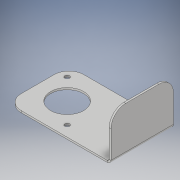
# Autodesk Inventor part: frontMotorMount
Saved by Autodesk Inventor 2017 (Build 210142000, 142)
## iProperties
Created: 2017-03-21
Part Number: frontMotorMount
Material: Generic
Document SubType Name: Sheet Metal
Designer: kingb
Density: 1 g/cm^3
Sheet Metal Rule: Default
Appearance: Default
Flat Pattern Width: 5.3975 cm
Flat Pattern Length: 12.7 cm
Flat Pattern Area: 68.5482 cm^2
Sheet Metal Width: 2.125 in
Sheet Metal Length: 5.000 in
Sheet Metal Area: 10.625 in^2
Author: kingb
Autodesk Inventor part; units mm, degrees
ref_plane "YZ Plane" through (0, 0, 0) normal (1, 0, 0) x (0, 1, 0)
ref_plane "XZ Plane" through (0, 0, 0) normal (0, 1, 0) x (-1, 0, 0)
ref_plane "XY Plane" through (0, 0, 0) normal (0, 0, 1) x (1, 0, 0)
sketch "Sketch1" plane through (0, 0, 0) normal (0, 1, 0) x (-1, 0, 0)
  line L0 (0, 0) -> (127, 0)
  line L1 (127, 0) -> (127, -53.975)
  line L2 (127, -53.975) -> (0, -53.975)
  line L3 (0, -53.975) -> (0, 0)
  line L4 (38.1, -53.975) -> (38.1, 0) construction
  line L5 (38.1, -26.9875) -> (101.6, -26.9875) construction
  circle A0 centre (101.6, -26.9875) radius 14.2875
  dimension "d0" = 127
  dimension "d1" = 53.975
  dimension "d2" = 38.1
  dimension "d3" = 63.5
  dimension "d4" = 28.575
  measures "d0" distance of L1.end L2.end
  measures "d1" distance of L0.end L1.end
  measures "d2" distance between parallel lines of L3 L4
  measures "d3" distance of L5.start L5.end
  measures "d4" diameter of A0
extrude "Plate1" add sketch "Sketch1" along normal blind 1.5875
fillet "Corner Round1" radius 12.7 2 edges at (-127, 0.7937, -53.975) (-127, 0.7937, 0)
fillet "Corner Round2" radius 12.7 2 edges at (0, 0.7937, 0) (0, 0.7937, -53.975)
sketch "Sketch2" plane through (0, 1.5875, 0) normal (0, 1, 0) x (1, 0, 0)
  circle A0 centre (-83.6395, 9.027) radius 2.0193 projected
  circle A1 centre (-119.5605, 44.948) radius 2.0193 projected
  point P0 (0, 0)
extrude "Extrusion1" cut sketch "Sketch2" against normal up to next
sketch "Sketch3" plane through (0, 1.5875, 0) normal (0, 1, 0) x (1, 0, 0)
  line L0 (0, 0) -> (-38.1, 0) construction
  line L1 (-12.7, 0) -> (-114.3, 0) construction
  line L2 (-38.1, 0) -> (-38.1, 53.975)
  line L3 (-114.3, 53.975) -> (-12.7, 53.975) projected
  dimension "d10" = 38.1
  constraints: 4 end point, 2 point on line, 1 perpendicular
  measures "d10" distance of L0.start L0.end
fold "Fold1" angle 90 bend radius 1.5875 thickness 1.5875 k factor 0.44 line from (-38.1, 1.5875, 0) to (-38.1, 1.5875, -53.975) line at bend centre moving side (1, 0, 0) folds toward (0, 1, 0)
equation "\"d11\" = BendReliefWidth"
equation "\"d12\" = BendReliefDepth"
equation "\"d13\" = MinimumRemnant"
equation "\"d14\" = BendRadius"
equation "\"d16\" = BendRadius"
equation "\"BendRadius\" = Thickness"
equation "\"BendReliefWidth\" = Thickness"
equation "\"BendReliefDepth\" = 0.5 * Thickness"
equation "\"CornerReliefSize\" = 4 * Thickness"
equation "\"MinimumRemnant\" = 2 * Thickness"
equation "\"TransitionRadius\" = BendRadius"
equation "\"JacobiRadiusSize\" = Thickness"
equation "\"GapSize\" = Thickness"
equation "\"d5\" = BendRadius"
equation "\"Thickness\" = 1.5875"
body "Solid1"
